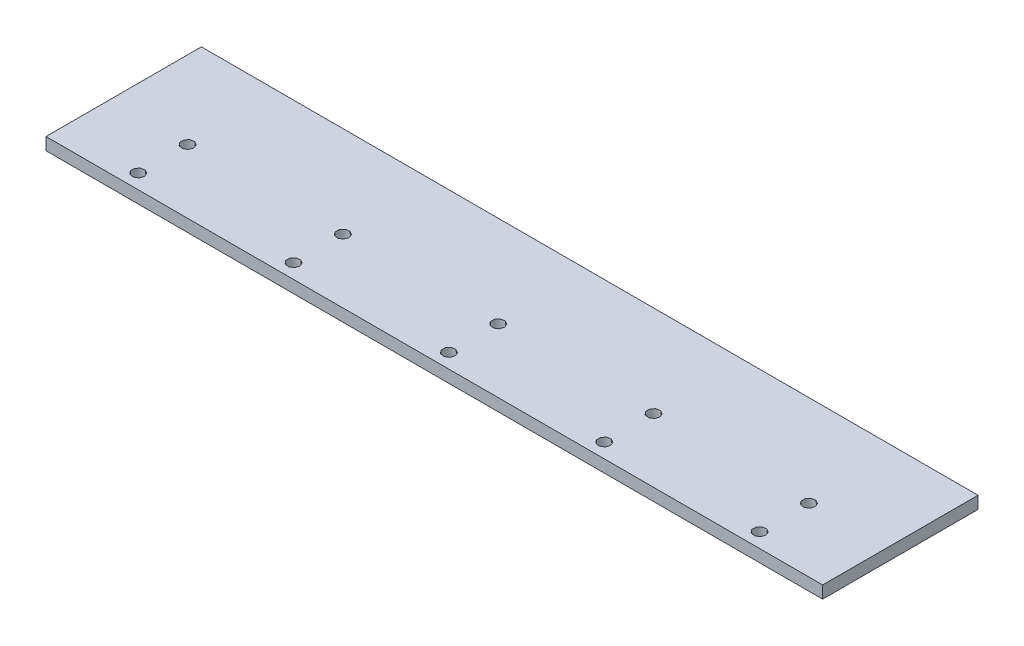
# Autodesk Inventor part: y_axis_mounting_plate
Saved by Autodesk Inventor 2014 (Build 180170000, 170)
## iProperties
Created: 2014-08-13
Part Number: y_axis_mounting_plate
Material: Generic
Document SubType Name: Modeling
Designer: Matthew
Density: 1 g/cm^3
Appearance: Default
Author: Matthew
Autodesk Inventor part; units mm, degrees
ref_plane "YZ Plane" through (0, 0, 0) normal (1, 0, 0) x (0, 1, 0)
ref_plane "XZ Plane" through (0, 0, 0) normal (0, 1, 0) x (-1, 0, 0)
ref_plane "XY Plane" through (0, 0, 0) normal (0, 0, 1) x (1, 0, 0)
sketch "Sketch1" plane through (0, 0, 0) normal (0, 1, 0) x (-1, 0, 0)
  line L0 (200, 40.005) -> (-200, 40.005)
  line L1 (-200, 40.005) -> (-200, -40.005)
  line L2 (-200, -40.005) -> (200, -40.005)
  line L3 (200, -40.005) -> (200, 40.005)
  line L4 (200, 40.005) -> (-200, -40.005) construction
  line L5 (-200, 40.005) -> (200, -40.005) construction
  point P0 (0, 0)
  dimension "d0" = 400
  dimension "d1" = 80.01
  constraints: 12 end point, 2 midpoint, 2 parallel, 1 horizontal, 1 perpendicular
  measures "d0" distance of L2.end L1.end
  measures "d1" distance of L2.end L0.start
extrude "Extrusion1" add sketch "Sketch1" along normal blind 6.35
sketch "Sketch2" plane through (0, 6.35, 0) normal (0, 1, 0) x (1, 0, 0)
  line L0 (-200, -40.005) -> (200, -40.005) projected
  line L1 (200, -40.005) -> (200, 40.005) projected
  line L2 (200, 40.005) -> (-200, 40.005) projected
  line L3 (-200, 40.005) -> (-200, -40.005) projected
  line L4 (-200, 18.3007) -> (200, 18.3007) construction
  point P0 (-200, 0.005)
  point P1 (-200, -7.0993)
  point P2 (-160, -7.0993)
  point P3 (-80, -7.0993)
  point P4 (0, -7.0993)
  point P5 (80, -7.0993)
  point P6 (160, -7.0993)
  point P7 (-160, -32.4993)
  point P8 (-80, -7.0993)
  point P9 (-80, -32.4993)
  point P10 (0, -7.0993)
  point P11 (0, -32.4993)
  point P12 (80, -7.0993)
  point P13 (80, -32.4993)
  point P14 (160, -7.0993)
  point P15 (160, -32.4993)
  dimension "d4" = 21.7043
  dimension "d5" = 40
  dimension "d6" = 25.4
  dimension "d7" = 40
  dimension "d24" = 25.4
  dimension "d27" = 80
  constraints: 4 point on line, 2 end point, 1 horizontal, 1 horizontal alignment, 1 parallel, 1 vertical, 9 other
  measures "d4" distance between parallel lines of L2 L4
  measures "d5" distance from line of L2 point (-200, 0.005)
  measures "d6" distance of L4.start point (-200, -7.099)
  measures "d7" distance from line of L3 point (-160, -7.099)
  measures "d24" distance of point (-160, -7.099) point (-160, -32.499)
  measures "d27" distance of point (-160, -7.099) point (-80, -7.099)
hole "Hole2" at (-160, 6.35, 7.0993) at (-80, 6.35, 7.0993) at (0, 6.35, 7.0993) at (80, 6.35, 7.0993) at (160, 6.35, 7.0993) at (-160, 6.35, 32.4993) at (-80, 6.35, 32.4993) at (0, 6.35, 32.4993) at (80, 6.35, 32.4993) at (160, 6.35, 32.4993) direction (0, -1, 0) diameter 6.35 depth 25.4 tip angle 118
body "Solid1"
